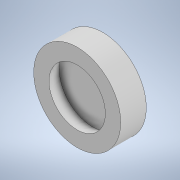
# Autodesk Inventor part: circle-reed
Saved by Autodesk Inventor 2021 (Build 250183000, 183)
## iProperties
Created: 2021-01-16
Part Number: circle-reed
Material: Generic
Document SubType Name: Modeling
Designer: Luke Kamols
Density: 1 g/cm^3
Appearance: Default
Author: Luke Kamols
Autodesk Inventor part; units mm, degrees
ref_plane "YZ Plane" through (0, 0, 0) normal (1, 0, 0) x (0, 1, 0)
ref_plane "XZ Plane" through (0, 0, 0) normal (0, 1, 0) x (-1, 0, 0)
ref_plane "XY Plane" through (0, 0, 0) normal (0, 0, 1) x (1, 0, 0)
sketch "Sketch1" plane through (0, 0, 0) normal (0, 1, 0) x (-1, 0, 0)
  line L0 (0, 0) -> (-5.5, 0)
  line L1 (-6.5, -3) -> (-5.5, 0)
  line L2 (-6.5, -3) -> (-8.5, -3)
  line L3 (-8.5, -3) -> (-8.5, 0)
  line L4 (-8.5, 0) -> (-5.5, 0)
  line L5 (0, 0) -> (0, -4.1468)
  dimension "d11" = 2
  constraints: 12 end point, 2 horizontal, 2 perpendicular, 1 vertical
  measures "d11" distance of L1.start L2.end
revolve "Revolution1" add sketch "Sketch1" angle 360 about axis through (0, 0, 0) along (0, 0, -1)
sketch "Sketch3" plane through (0, 0, -3) normal (0, 0, -1) x (-1, 0, 0)
  circle A0 centre (0, 0) radius 8.5 projected
extrude "Extrusion3" add sketch "Sketch3" along normal blind 2
body "Solid2"
